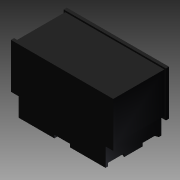
# Autodesk Inventor part: 03
Saved by Autodesk Inventor 2012 (Build 160160000, 160)
## iProperties
Created: 2014-01-27
Part Number: 03
Material: Default
Document SubType Name: Modeling
Designer: Michał
Density: 1 g/cm^3
Author: Michał
Autodesk Inventor part; units mm, degrees
ref_plane "YZ Plane" through (0, 0, 0) normal (1, 0, 0) x (0, 1, 0)
ref_plane "XZ Plane" through (0, 0, 0) normal (0, 1, 0) x (-1, 0, 0)
sketch "Sketch1" plane through (0, 0, 0) normal (0, 0, 1) x (1, 0, 0)
  line L0 (-16, -8) -> (16, -8)
  line L1 (16, -8) -> (16, 8)
  line L2 (16, 8) -> (-16, 8)
  line L3 (-16, 8) -> (-16, -8)
  point P0 (0, 0)
  point P1 (0, 8)
  point P2 (16, 0)
  dimension "d0" = 32
  dimension "d1" = 16
  constraints: 8 end point, 2 midpoint, 2 parallel, 1 horizontal, 1 horizontal alignment, 1 perpendicular, 1 vertical alignment
  measures "d0" distance of L2.end L1.end
  measures "d1" distance of L1.end L0.end
extrude "Extrusion1" add sketch "Sketch1" along normal blind 13
sketch "Sketch2" plane through (-16, -8, 0) normal (0, -1, 0) x (1, 0, 0)
  line L0 (32, 13) -> (0, 13) projected
  line L1 (0, 0) -> (0, 13) projected
  line L2 (0, 0) -> (32, 0) projected
  line L3 (32, 0) -> (32, 13) projected
  line L4 (-1, 14) -> (33, 14)
  line L5 (33, 14) -> (33, -1)
  line L6 (33, -1) -> (-1, -1)
  line L7 (-1, -1) -> (-1, 14)
  line L8 (2, -1) -> (30, -1)
  line L9 (30, -1) -> (30, -7)
  line L10 (30, -7) -> (2, -7)
  line L11 (2, -7) -> (2, -1)
  point P0 (16, 0)
  dimension "d4" = 1
  dimension "d5" = 3
  dimension "d6" = 3
  dimension "d7" = 6
  constraints: 16 end point, 2 parallel, 1 horizontal, 1 perpendicular, 1 point on line, 3 other
  measures "d4" distance between parallel lines of L4 L0
  measures "d5" distance between parallel lines of L7 L11
  measures "d6" distance between parallel lines of L5 L9
  measures "d7" distance between parallel lines of L6 L10
extrude "Extrusion2" add sketch "Sketch2" along normal blind 1 contours L3 L2 L1 L0 | L4 L5 L6 L7 | L6 L9 L10 L11
sketch "Sketch3" plane through (-16, -8, 0) normal (0, 1, 0) x (1, 0, 0)
  line L0 (0, 0) -> (32, 0) projected
  line L1 (2, 7) -> (30, 7)
  line L2 (30, 7) -> (30, 0)
  line L3 (30, 0) -> (2, 0)
  line L4 (2, 0) -> (2, 7)
  point P0 (16, 0)
  constraints: 8 end point, 2 parallel, 1 horizontal, 1 perpendicular, 1 point on line
extrude "Extrusion3" add sketch "Sketch3" along normal up to surface (16 mm away)
sketch "Sketch4" plane through (-16, 8, 13) normal (0, 1, 0) x (1, 0, 0)
  line L0 (0, 0) -> (32, 0) projected
  line L1 (32, 13) -> (32, 0) projected
  line L2 (32, 13) -> (30, 13) projected
  line L3 (30, 20) -> (30, 13) projected
  line L4 (2, 20) -> (30, 20) projected
  line L5 (2, 13) -> (2, 20) projected
  line L6 (2, 13) -> (0, 13) projected
  line L7 (0, 13) -> (0, 0) projected
  line L8 (-1, 14) -> (2, 14) projected
  line L9 (2, 13) -> (2, 14) projected
  line L10 (-1, 14) -> (2, 14) projected
  line L11 (-1, -1) -> (-1, 14) projected
  line L12 (33, -1) -> (-1, -1) projected
  line L13 (33, 14) -> (33, -1) projected
  line L14 (30, 14) -> (33, 14) projected
  line L15 (30, 14) -> (30, 13) projected
  line L16 (30, 13) -> (32, 13) projected
  line L17 (32, 13) -> (32, 0) projected
  line L18 (32, 0) -> (0, 0) projected
  line L19 (0, 13) -> (0, 0) projected
  line L20 (0, 13) -> (2, 13) projected
  point P0 (16, 13)
extrude "Extrusion4" add sketch "Sketch4" along normal blind 1
sketch "Sketch5" plane through (14, -9, -7) normal (0, 0, -1) x (-1, 0, 0)
  line L0 (28, 0) -> (28, 18) projected
  line L1 (28, 18) -> (0, 18) projected
  line L2 (0, 18) -> (0, 0) projected
  line L3 (11.5, 18) -> (16.5, 18)
  line L4 (16.5, 18) -> (16.5, 13)
  line L5 (16.5, 13) -> (11.5, 13)
  line L6 (11.5, 13) -> (11.5, 18)
  circle A0 centre (14, 13) radius 2.5
  circle A1 centre (23, 13) radius 2.5
  line L7 (23.7463, 10.614) -> (28, 11.9446)
  line L8 (22.2537, 15.386) -> (28, 17.1835)
  circle A2 centre (5, 13) radius 2.5
  line L9 (4.2537, 10.614) -> (0, 11.9446)
  line L10 (5.7463, 15.386) -> (0, 17.1835)
  point P0 (14, 9)
  point P1 (14, 18)
  point P2 (14, 18)
  dimension "d14" = 5
  dimension "d15" = 5
  dimension "d16" = 5
  dimension "d17" = 9
  dimension "d18" = 5
  dimension "d19" = 9
  constraints: 16 end point, 5 point on line, 4 parallel, 4 point on circle, 4 tangent, 3 midpoint, 2 centre point, 1 coincident, 1 horizontal, 1 horizontal alignment, 1 perpendicular, 2 other
  measures "d14" distance of L4.end L5.end
  measures "d15" distance of L3.end L4.end
  measures "d16" diameter of A1
  measures "d17" distance of point (14, 13) A1.centre
  measures "d18" diameter of A2
  measures "d19" distance of A2.centre point (14, 13)
extrude "Extrusion5" cut sketch "Sketch5" against normal blind 1
ref_plane "Work Plane1" through (-16, 0, 13) normal (0, 1, 0) x (1, 0, 0)
mirror "Mirror1" about plane through (-16, 0, 13) normal (0, 1, 0) of "Extrusion5"
sketch "Sketch6" plane through (-17, -8, 14) normal (0, 0, 1) x (1, 0, 0)
  line L0 (0, -1) -> (34, -1) projected
  line L1 (34, 0) -> (34, -1) projected
  line L2 (34, 0) -> (0, 0) projected
  line L3 (0, 0) -> (0, -1) projected
  line L4 (34, 17) -> (0, 17) projected
  line L5 (0, 16) -> (0, 17) projected
  line L6 (0, 16) -> (34, 16) projected
  line L7 (34, 16) -> (34, 17) projected
  point P0 (17, 8)
extrude "Extrusion6" cut sketch "Sketch6" against normal blind 0.5
sketch "Sketch7" plane through (17, -9, -1) normal (1, 0, 0) x (0, 0, -1)
  line L0 (-14.5, 1) -> (-14.5, 0) projected
  line L1 (-14.5, 0) -> (0, 0) projected
  line L2 (0, 1) -> (0, 0) projected
  line L3 (0, 1) -> (-14.5, 1) projected
  line L4 (-14.5, 18) -> (-14.5, 17) projected
  line L5 (-14.5, 17) -> (0, 17) projected
  line L6 (0, 17) -> (0, 18) projected
  line L7 (0, 18) -> (-14.5, 18) projected
  point P0 (-1, 9)
extrude "Extrusion7" cut sketch "Sketch7" against normal blind 0.5
sketch "Sketch8" plane through (-17, 8, -1) normal (-1, 0, 0) x (0, 0, 1)
  line L0 (14.5, 0) -> (14.5, 1) projected
  line L1 (14.5, 1) -> (0, 1) projected
  line L2 (0, 0) -> (0, 1) projected
  line L3 (0, 0) -> (14.5, 0) projected
  line L4 (14.5, -17) -> (14.5, -16) projected
  line L5 (14.5, -16) -> (0, -16) projected
  line L6 (0, -16) -> (0, -17) projected
  line L7 (0, -17) -> (14.5, -17) projected
  point P0 (1, -8)
extrude "Extrusion8" cut sketch "Sketch8" against normal blind 0.5
equation "\"d6\" = d5"
body "Solid1"
